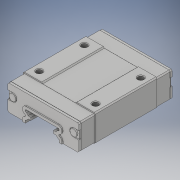
# Autodesk Inventor part: SSEBZ-MX16_b
Saved by Autodesk Inventor 2019 (Build 230136000, 136)
## iProperties
Created: 2022-12-29
Part Number: SSEBZ-MX16_b
Material: Generic
Catalog Web Link: www.cadenas.de
Description: SSEBZ, SSEBZ-MX, SSE2BZ, SSE2BZ-MX, SSEBLZ, SSEBLZ-MX, SSE2BLZ, SSE2BLZ-MX, SEBZ, SE2BZ, SEBLZ, SE2BLZ_block-Miniature Linear Guides - Standard Blocks - Light Preload/Slight Clearance - Standard Grade - Selectable/Configurable
Vendor: MISUMI
Document SubType Name: Modeling
Designer: psAdmin
Manufacturer: MISUMI
Mass: 12.2418 g
Surface Area: 52.4298 cm^2
Volume: 12.2418 cm^3
Density: 1 g/cm^3
Appearance: PSOLRGB-175-175-175
Category: PARTsolutions
Company: MISUMI
Title: SSEBZ-MX16
Author: Cadenas PARTsolutions
Comments: Miniature Linear Guides - Standard Blocks - Light Preload/Slight Clearance - Standard Grade - Selectable/Configurable
PSOL_IDENT_0: {$CADENAS_DATA/23d-libs/misumi/metric/06_linear_guides/ssebz_series/sebz_block.prj},271 {VTYP=3D},{N
PSOL_IDENT_1: B=SSEBZ-MX16_b},{LINA=SSEBZ-MX16},{NN=SSEBZ, SSEBZ-MX, SSE2BZ, SSE2BZ-MX, SSEBLZ, SSEBLZ-MX, SSE2BLZ
PSOL_IDENT_2: , SSE2BLZ-MX, SEBZ, SE2BZ, SEBLZ, SE2BLZ_block},{DATE=01.06.2021 05:33:22},{GEOMDATE=29.09.2020 01:4
PSOL_IDENT_3: 8:00},{VERSION=},{LINEID=300},{WBVAR=MAT,MX},{WBNUMERIC=}  {NB=SSEBZ-MX16_b},{LINA=SSEBZ-MX16},{KT=D
PSOL_IDENT_4: UMMY},{PN=SSEBZ-MX16},{TS=Z},{TYPE=SSEBZ},{H=16},{MAT=S},{MX=-MX},{MXALG='', 'w/o MX(Lubrication uni
PSOL_IDENT_5: t)', '-MX', 'with MX(Lubrication unit)'},{W=32},{L1=42.4},{B=25},{C=20},{SLL=M3x4},{S=3},{LL=4.0},{L
PSOL_IDENT_6: 2=27.4},{K=12.0},{CBB=0.5},{W1=15},{W2=8.5},{H1=9.5},{CAA=0.5},{F=40},{G=15.0},{CA1=0.3},{CA2=0.5},{
PSOL_IDENT_7: VA1=2.5},{HA1=2.5},{WA1=3.4477},{WA2=1.2},{RA1=3.50},{HA2=15.6300},{POIA1=0.2300},{BHA1=27.0},{BHA2=
PSOL_IDENT_8: 31.5},{BHA3=31.6},{BHA5=17.9450},{BHA6=31.1},{BHA7=14.6},{BHA8=7.4},{BVA1=5.20},{BVA3=0.50},{BVA4=0.
PSOL_IDENT_9: 60},{BVA5=11.30},{BVA6=11.40},{BCA1=0.5},{BCA2H=0.5},{BCA2V=0.45},{BRA1=1.80},{BRA2=1.50},{BDA1=25.0
PSOL_IDENT_10: 0},{BHB1=17.4600},{BHB2=15.5484},{BVB1=6.6300},{BVB2=3.5286},{BRB1=1.6},{BRB2=1.3000},{BRB3=0.4},{BH
PSOL_IDENT_11: C1=6.00},{BHC2=1.0},{BHC3=0.6},{BHC4=0.4},{BHC5=0.5},{MD=7.0}
NB: SSEBZ-MX16_b
NN: SSEBZ, SSEBZ-MX, SSE2BZ, SSE2BZ-MX, SSEBLZ, SSEBLZ-MX, SSE2BLZ, SSE2BLZ-MX, SEBZ, SE2BZ, SEBLZ, SE2BLZ_block
NT: Miniature Linear Guides - Standard Blocks - Light Preload/Slight Clearance - Standard Grade - Selectable/Configurable
NBSYN: $PN._b
LINA: SSEBZ-MX16
CATALOG: Misumi
PN: SSEBZ-MX16
H: 16
MAT: Stainless Steel
MX: with MX(Lubrication unit)
W: 32
L1: 42.4
B: 25
C: 20
SLL: M3x4
S: 3
LL: 4
L2: 27.4
K: 12
CBB: 0.5
W1: 15
W2: 8.5
H1: 9.5
CAA: 0.5
F: 40
G: 15
CA1: 0.3
CA2: 0.5
VA1: 2.5
HA1: 2.5
WA1: 3.4477
WA2: 1.2
RA1: 3.5
HA2: 15.63
POIA1: 0.23
BHA1: 27
BHA2: 31.5
BHA3: 31.6
BHA5: 17.945
BHA6: 31.1
BHA7: 14.6
BHA8: 7.4
BVA1: 5.2
BVA3: 0.5
BVA4: 0.6
BVA5: 11.3
BVA6: 11.4
BCA1: 0.5
BCA2H: 0.5
BCA2V: 0.45
BRA1: 1.8
BRA2: 1.5
BDA1: 25
BHB1: 17.46
BHB2: 15.5484
BVB1: 6.63
BVB2: 3.5286
BRB1: 1.6
BRB2: 1.3
BRB3: 0.4
BHC1: 6
BHC2: 1
BHC3: 0.6
BHC4: 0.4
BHC5: 0.5
MD: 7
SUPPLIER: MISUMI
ARTICLENO: SSEBZ-MX16_b
BOMINFO: SSEBZ-MX16
CREATOR: CADENAS GmbH
Autodesk Inventor part; units mm, degrees
sketch "Sketch_2" plane through (0, 0, 0) normal (0, 0, 1) x (1, 0, 0)
  line L0 (-16, 4.5) -> (-15.5, 4)
  line L1 (-15.5, 4) -> (-8.9725, 4)
  line L2 (-8.9725, 4) -> (-8.758, 4.1)
  line L3 (-8.758, 4.1) -> (8.758, 4.1)
  line L4 (8.758, 4.1) -> (8.9725, 4)
  line L5 (8.9725, 4) -> (15.5, 4)
  line L6 (15.5, 4) -> (16, 4.5)
  line L7 (16, 4.5) -> (16, 15.5)
  line L8 (16, 15.5) -> (15.5, 16)
  line L9 (15.5, 16) -> (7.8, 16)
  line L10 (7.8, 16) -> (7.3, 15.55)
  line L11 (7.3, 15.55) -> (-7.3, 15.55)
  line L12 (-7.3, 15.55) -> (-7.8, 16)
  line L13 (-7.8, 16) -> (-15.5, 16)
  line L14 (-15.5, 16) -> (-16, 15.5)
  line L15 (-16, 15.5) -> (-16, 4.5)
  constraints: 32 end point
extrude "Extrusion1" add sketch "Sketch_2" along normal mid plane 27.4
sketch "Sketch_3" plane through (0, 0, 13.7) normal (0, 0, 1) x (1, 0, 0)
  line L0 (-15.8, 15) -> (-15.8, 4.6)
  line L1 (-15.8, 4.6) -> (-15.3, 4.1)
  line L2 (-15.3, 4.1) -> (15.3, 4.1)
  line L3 (15.3, 4.1) -> (15.8, 4.6)
  line L4 (15.8, 4.6) -> (15.8, 15)
  line L5 (15.8, 15) -> (15.3, 15.5)
  line L6 (15.3, 15.5) -> (-15.3, 15.5)
  line L7 (-15.3, 15.5) -> (-15.8, 15)
  constraints: 16 end point
extrude "Extrusion2" add sketch "Sketch_3" along normal blind 7.5
sketch "Sketch_4" plane through (0, 0, -13.7) normal (0, 0, 1) x (1, 0, 0)
  line L0 (-15.8, 15) -> (-15.8, 4.6)
  line L1 (-15.8, 4.6) -> (-15.3, 4.1)
  line L2 (-15.3, 4.1) -> (15.3, 4.1)
  line L3 (15.3, 4.1) -> (15.8, 4.6)
  line L4 (15.8, 4.6) -> (15.8, 15)
  line L5 (15.8, 15) -> (15.3, 15.5)
  line L6 (15.3, 15.5) -> (-15.3, 15.5)
  line L7 (-15.3, 15.5) -> (-15.8, 15)
  constraints: 16 end point
extrude "Extrusion3" add sketch "Sketch_4" against normal blind 7.5
sketch "Sketch_8" plane through (0, 0, 21.2) normal (0, 0, 1) x (1, 0, 0)
  line L0 (-32, 24) -> (-32, 0)
  line L1 (-32, 0) -> (32, 0)
  line L2 (32, 0) -> (32, 24)
  line L3 (32, 24) -> (-32, 24)
  line L4 (-15.75, 12.6) -> (-13.5, 12.6)
  arc A0 (-13.5, 9) -> (-13.5, 12.6) centre (-13.5, 10.8) ccw
  line L5 (-13.5, 9) -> (-15.75, 9)
  line L6 (-15.75, 9) -> (-15.75, 4.6)
  line L7 (-15.75, 4.6) -> (-15.25, 4.1)
  line L8 (-15.25, 4.1) -> (15.25, 4.1)
  line L9 (15.25, 4.1) -> (15.75, 4.6)
  line L10 (15.75, 4.6) -> (15.75, 9)
  line L11 (15.75, 9) -> (13.5, 9)
  arc A1 (13.5, 12.6) -> (13.5, 9) centre (13.5, 10.8) ccw
  line L12 (13.5, 12.6) -> (15.75, 12.6)
  line L13 (15.75, 12.6) -> (15.75, 14.9)
  line L14 (15.75, 14.9) -> (15.25, 15.4)
  line L15 (15.25, 15.4) -> (-15.25, 15.4)
  line L16 (-15.25, 15.4) -> (-15.75, 14.9)
  line L17 (-15.75, 14.9) -> (-15.75, 12.6)
  constraints: 36 end point, 4 point on circle, 2 centre point
extrude "Extrusion4" cut sketch "Sketch_8" against normal blind 1.5
sketch "Sketch_15" plane through (0, 0, 21.2) normal (0, 0, 1) x (1, 0, 0)
  line L0 (-32, 24) -> (-32, 0)
  line L1 (-32, 0) -> (32, 0)
  line L2 (32, 0) -> (32, 24)
  line L3 (32, 24) -> (-32, 24)
  line L4 (-8.73, 4.1) -> (8.73, 4.1)
  line L5 (8.73, 4.1) -> (8.73, 5.2357)
  arc A0 (8.73, 5.2357) -> (8.0801, 6.3615) centre (7.43, 5.2357) ccw
  line L6 (8.0801, 6.3615) -> (7.5742, 6.6536)
  arc A1 (7.5742, 7.3464) -> (7.5742, 6.6536) centre (7.7742, 7) ccw
  line L7 (7.5742, 7.3464) -> (8.0801, 7.6385)
  arc A2 (8.0801, 7.6385) -> (8.73, 8.7643) centre (7.43, 8.7643) ccw
  line L8 (8.73, 8.7643) -> (8.73, 9.13)
  arc A3 (8.73, 9.13) -> (7.13, 10.73) centre (7.13, 9.13) ccw
  line L9 (7.13, 10.73) -> (-7.13, 10.73)
  arc A4 (-7.13, 10.73) -> (-8.73, 9.13) centre (-7.13, 9.13) ccw
  line L10 (-8.73, 9.13) -> (-8.73, 8.7643)
  arc A5 (-8.73, 8.7643) -> (-8.0801, 7.6385) centre (-7.43, 8.7643) ccw
  line L11 (-8.0801, 7.6385) -> (-7.5742, 7.3464)
  arc A6 (-7.5742, 6.6536) -> (-7.5742, 7.3464) centre (-7.7742, 7) ccw
  line L12 (-7.5742, 6.6536) -> (-8.0801, 6.3615)
  arc A7 (-8.0801, 6.3615) -> (-8.73, 5.2357) centre (-7.43, 5.2357) ccw
  line L13 (-8.73, 5.2357) -> (-8.73, 4.1)
  constraints: 28 end point, 16 point on circle, 8 centre point
extrude "Extrusion5" cut sketch "Sketch_15" against normal blind 0.5
sketch "Sketch_7" plane through (0, 0, -21.2) normal (0, 0, 1) x (1, 0, 0)
  line L0 (-32, 24) -> (-32, 0)
  line L1 (-32, 0) -> (32, 0)
  line L2 (32, 0) -> (32, 24)
  line L3 (32, 24) -> (-32, 24)
  line L4 (-15.75, 12.6) -> (-13.5, 12.6)
  arc A0 (-13.5, 9) -> (-13.5, 12.6) centre (-13.5, 10.8) ccw
  line L5 (-13.5, 9) -> (-15.75, 9)
  line L6 (-15.75, 9) -> (-15.75, 4.6)
  line L7 (-15.75, 4.6) -> (-15.25, 4.1)
  line L8 (-15.25, 4.1) -> (15.25, 4.1)
  line L9 (15.25, 4.1) -> (15.75, 4.6)
  line L10 (15.75, 4.6) -> (15.75, 9)
  line L11 (15.75, 9) -> (13.5, 9)
  arc A1 (13.5, 12.6) -> (13.5, 9) centre (13.5, 10.8) ccw
  line L12 (13.5, 12.6) -> (15.75, 12.6)
  line L13 (15.75, 12.6) -> (15.75, 14.9)
  line L14 (15.75, 14.9) -> (15.25, 15.4)
  line L15 (15.25, 15.4) -> (-15.25, 15.4)
  line L16 (-15.25, 15.4) -> (-15.75, 14.9)
  line L17 (-15.75, 14.9) -> (-15.75, 12.6)
  constraints: 36 end point, 4 point on circle, 2 centre point
extrude "Extrusion6" cut sketch "Sketch_7" along normal blind 1.5
sketch "Sketch_13" plane through (0, 0, -21.2) normal (0, 0, 1) x (1, 0, 0)
  line L0 (-32, 24) -> (-32, 0)
  line L1 (-32, 0) -> (32, 0)
  line L2 (32, 0) -> (32, 24)
  line L3 (32, 24) -> (-32, 24)
  line L4 (-8.73, 4.1) -> (8.73, 4.1)
  line L5 (8.73, 4.1) -> (8.73, 5.2357)
  arc A0 (8.73, 5.2357) -> (8.0801, 6.3615) centre (7.43, 5.2357) ccw
  line L6 (8.0801, 6.3615) -> (7.5742, 6.6536)
  arc A1 (7.5742, 7.3464) -> (7.5742, 6.6536) centre (7.7742, 7) ccw
  line L7 (7.5742, 7.3464) -> (8.0801, 7.6385)
  arc A2 (8.0801, 7.6385) -> (8.73, 8.7643) centre (7.43, 8.7643) ccw
  line L8 (8.73, 8.7643) -> (8.73, 9.13)
  arc A3 (8.73, 9.13) -> (7.13, 10.73) centre (7.13, 9.13) ccw
  line L9 (7.13, 10.73) -> (-7.13, 10.73)
  arc A4 (-7.13, 10.73) -> (-8.73, 9.13) centre (-7.13, 9.13) ccw
  line L10 (-8.73, 9.13) -> (-8.73, 8.7643)
  arc A5 (-8.73, 8.7643) -> (-8.0801, 7.6385) centre (-7.43, 8.7643) ccw
  line L11 (-8.0801, 7.6385) -> (-7.5742, 7.3464)
  arc A6 (-7.5742, 6.6536) -> (-7.5742, 7.3464) centre (-7.7742, 7) ccw
  line L12 (-7.5742, 6.6536) -> (-8.0801, 6.3615)
  arc A7 (-8.0801, 6.3615) -> (-8.73, 5.2357) centre (-7.43, 5.2357) ccw
  line L13 (-8.73, 5.2357) -> (-8.73, 4.1)
  constraints: 28 end point, 16 point on circle, 8 centre point
extrude "Extrusion7" cut sketch "Sketch_13" along normal blind 0.5
sketch "Sketch_25" plane through (0, 0, 19.7) normal (0, 0, 1) x (1, 0, 0)
  line L0 (-15.55, 12.6) -> (-15.55, 9)
  line L1 (-15.55, 9) -> (-13.5, 9)
  arc A0 (-13.5, 9) -> (-13.5, 12.6) centre (-13.5, 10.8) ccw
  line L2 (-13.5, 12.6) -> (-15.55, 12.6)
  constraints: 6 end point, 2 point on circle, 1 centre point
extrude "Extrusion8" add sketch "Sketch_25" along normal blind 0.6
sketch "Sketch_5" plane through (0, 0, 19.7) normal (0, 0, 1) x (1, 0, 0)
  arc A0 (13.5, 12.6) -> (13.5, 9) centre (13.5, 10.8) ccw
  line L0 (13.5, 9) -> (15.55, 9)
  line L1 (15.55, 9) -> (15.55, 12.6)
  line L2 (15.55, 12.6) -> (13.5, 12.6)
  constraints: 6 end point, 2 point on circle, 1 centre point
extrude "Extrusion9" add sketch "Sketch_5" along normal blind 0.6
sketch "Sketch_9" plane through (0, 0, -19.7) normal (0, 0, 1) x (1, 0, 0)
  line L0 (-15.55, 12.6) -> (-15.55, 9)
  line L1 (-15.55, 9) -> (-13.5, 9)
  arc A0 (-13.5, 9) -> (-13.5, 12.6) centre (-13.5, 10.8) ccw
  line L2 (-13.5, 12.6) -> (-15.55, 12.6)
  constraints: 6 end point, 2 point on circle, 1 centre point
extrude "Extrusion10" add sketch "Sketch_9" against normal blind 0.6
sketch "Sketch_26" plane through (0, 0, -19.7) normal (0, 0, 1) x (1, 0, 0)
  arc A0 (13.5, 12.6) -> (13.5, 9) centre (13.5, 10.8) ccw
  line L0 (13.5, 9) -> (15.55, 9)
  line L1 (15.55, 9) -> (15.55, 12.6)
  line L2 (15.55, 12.6) -> (13.5, 12.6)
  constraints: 6 end point, 2 point on circle, 1 centre point
extrude "Extrusion11" add sketch "Sketch_26" against normal blind 0.6
sketch "Sketch_18" plane through (-13.5, 0, 0) normal (1, 0, 0) x (0, 0, -1)
  line L0 (-20.3, 10.8) -> (-20.9, 10.8)
  line L1 (-20.9, 10.8) -> (-20.9, 12.3)
  line L2 (-20.9, 12.3) -> (-20.3, 12.3)
  line L3 (-20.3, 12.3) -> (-20.3, 10.8)
  line L4 (-20.3, 10.8) -> (-20.9, 10.8)
  constraints: 10 end point
revolve "Revolution1" add sketch "Sketch_18" angle 360 about axis through (-13.5, 10.8, 20.3) along (0, 0, -1)
sketch "Sketch_19" plane through (-13.5, 0, 0) normal (1, 0, 0) x (0, 0, -1)
  line L0 (20.9, 10.8) -> (20.3, 10.8)
  line L1 (20.3, 10.8) -> (20.3, 12.3)
  line L2 (20.3, 12.3) -> (20.9, 12.3)
  line L3 (20.9, 12.3) -> (20.9, 10.8)
  line L4 (20.9, 10.8) -> (20.3, 10.8)
  constraints: 10 end point
revolve "Revolution2" add sketch "Sketch_19" angle 360 about axis through (-13.5, 10.8, -20.9) along (0, 0, -1)
sketch "Sketch_20" plane through (13.5, 0, 0) normal (1, 0, 0) x (0, 0, -1)
  line L0 (-20.3, 10.8) -> (-20.9, 10.8)
  line L1 (-20.9, 10.8) -> (-20.9, 12.3)
  line L2 (-20.9, 12.3) -> (-20.3, 12.3)
  line L3 (-20.3, 12.3) -> (-20.3, 10.8)
  line L4 (-20.3, 10.8) -> (-20.9, 10.8)
  constraints: 10 end point
revolve "Revolution3" add sketch "Sketch_20" angle 360 about axis through (13.5, 10.8, 20.3) along (0, 0, -1)
sketch "Sketch_21" plane through (13.5, 0, 0) normal (1, 0, 0) x (0, 0, -1)
  line L0 (20.9, 10.8) -> (20.3, 10.8)
  line L1 (20.3, 10.8) -> (20.3, 12.3)
  line L2 (20.3, 12.3) -> (20.9, 12.3)
  line L3 (20.9, 12.3) -> (20.9, 10.8)
  line L4 (20.9, 10.8) -> (20.3, 10.8)
  constraints: 10 end point
revolve "Revolution4" add sketch "Sketch_21" angle 360 about axis through (13.5, 10.8, -20.9) along (0, 0, -1)
sketch "Sketch_17" plane through (0, 0, 0) normal (0, 0, 1) x (1, 0, 0)
  line L0 (-7.5, 9.2) -> (-7.5, 8.7239)
  line L1 (-7.5, 8.7239) -> (-6.94, 8.4006)
  arc A0 (-6.2177, 7.6) -> (-6.94, 8.4006) centre (-7.815, 6.885) ccw
  line L2 (-6.2177, 7.6) -> (-5, 7.6)
  line L3 (-5, 7.6) -> (-5, 6.4)
  line L4 (-5, 6.4) -> (-6.2177, 6.4)
  arc A1 (-6.94, 5.5994) -> (-6.2177, 6.4) centre (-7.815, 7.115) ccw
  line L5 (-6.94, 5.5994) -> (-7.5, 5.2762)
  line L6 (-7.5, 5.2762) -> (-7.5, 0.5)
  line L7 (-7.5, 0.5) -> (-7, 0)
  line L8 (-7, 0) -> (7, 0)
  line L9 (7, 0) -> (7.5, 0.5)
  line L10 (7.5, 0.5) -> (7.5, 5.2762)
  line L11 (7.5, 5.2762) -> (6.94, 5.5994)
  arc A2 (6.2177, 6.4) -> (6.94, 5.5994) centre (7.815, 7.115) ccw
  line L12 (6.2177, 6.4) -> (5, 6.4)
  line L13 (5, 6.4) -> (5, 7.6)
  line L14 (5, 7.6) -> (6.2177, 7.6)
  arc A3 (6.94, 8.4006) -> (6.2177, 7.6) centre (7.815, 6.885) ccw
  line L15 (6.94, 8.4006) -> (7.5, 8.7239)
  line L16 (7.5, 8.7239) -> (7.5, 9.2)
  line L17 (7.5, 9.2) -> (7.2, 9.5)
  line L18 (7.2, 9.5) -> (-7.2, 9.5)
  line L19 (-7.2, 9.5) -> (-7.5, 9.2)
  constraints: 40 end point, 8 point on circle, 4 centre point
extrude "Extrusion12" cut sketch "Sketch_17" along normal mid plane 27.4
sketch "Sketch_11" plane through (0, 0, 13.7) normal (0, 0, 1) x (1, 0, 0)
  line L0 (-7.5, 9.2) -> (-7.5, 8.7239)
  line L1 (-7.5, 8.7239) -> (-6.94, 8.4006)
  arc A0 (-6.2177, 7.6) -> (-6.94, 8.4006) centre (-7.815, 6.885) ccw
  line L2 (-6.2177, 7.6) -> (-5, 7.6)
  line L3 (-5, 7.6) -> (-5, 6.4)
  line L4 (-5, 6.4) -> (-6.2177, 6.4)
  arc A1 (-6.94, 5.5994) -> (-6.2177, 6.4) centre (-7.815, 7.115) ccw
  line L5 (-6.94, 5.5994) -> (-7.5, 5.2762)
  line L6 (-7.5, 5.2762) -> (-7.5, 0.5)
  line L7 (-7.5, 0.5) -> (-7, 0)
  line L8 (-7, 0) -> (7, 0)
  line L9 (7, 0) -> (7.5, 0.5)
  line L10 (7.5, 0.5) -> (7.5, 5.2762)
  line L11 (7.5, 5.2762) -> (6.94, 5.5994)
  arc A2 (6.2177, 6.4) -> (6.94, 5.5994) centre (7.815, 7.115) ccw
  line L12 (6.2177, 6.4) -> (5, 6.4)
  line L13 (5, 6.4) -> (5, 7.6)
  line L14 (5, 7.6) -> (6.2177, 7.6)
  arc A3 (6.94, 8.4006) -> (6.2177, 7.6) centre (7.815, 6.885) ccw
  line L15 (6.94, 8.4006) -> (7.5, 8.7239)
  line L16 (7.5, 8.7239) -> (7.5, 9.2)
  line L17 (7.5, 9.2) -> (7.2, 9.5)
  line L18 (7.2, 9.5) -> (-7.2, 9.5)
  line L19 (-7.2, 9.5) -> (-7.5, 9.2)
  constraints: 40 end point, 8 point on circle, 4 centre point
extrude "Extrusion13" cut sketch "Sketch_11" along normal blind 13.7
sketch "Sketch_22" plane through (0, 0, 13.7) normal (0, 0, 1) x (1, 0, 0)
  line L0 (-32, 24) -> (-32, 0)
  line L1 (-32, 0) -> (32, 0)
  line L2 (32, 0) -> (32, 24)
  line L3 (32, 24) -> (-32, 24)
  line L4 (-15.8, 15.05) -> (-15.8, 4.55)
  line L5 (-15.8, 4.55) -> (-15.35, 4.1)
  line L6 (-15.35, 4.1) -> (-7.55, 4.1)
  line L7 (-7.55, 4.1) -> (-7.55, 5.3262)
  line L8 (-7.55, 5.3262) -> (-7.0074, 5.6191)
  arc A0 (-7.0074, 5.6191) -> (-6.2505, 6.45) centre (-7.815, 7.115) ccw
  line L9 (-6.2505, 6.45) -> (-5.05, 6.45)
  line L10 (-5.05, 6.45) -> (-5.05, 7.55)
  line L11 (-5.05, 7.55) -> (-6.2505, 7.55)
  arc A1 (-6.2505, 7.55) -> (-7.0074, 8.3809) centre (-7.815, 6.885) ccw
  line L12 (-7.0074, 8.3809) -> (-7.55, 8.6739)
  line L13 (-7.55, 8.6739) -> (-7.55, 9.25)
  line L14 (-7.55, 9.25) -> (-7.25, 9.55)
  line L15 (-7.25, 9.55) -> (7.25, 9.55)
  line L16 (7.25, 9.55) -> (7.55, 9.25)
  line L17 (7.55, 9.25) -> (7.55, 8.6739)
  line L18 (7.55, 8.6739) -> (7.0074, 8.3809)
  arc A2 (7.0074, 8.3809) -> (6.2505, 7.55) centre (7.815, 6.885) ccw
  line L19 (6.2505, 7.55) -> (5.05, 7.55)
  line L20 (5.05, 7.55) -> (5.05, 6.45)
  line L21 (5.05, 6.45) -> (6.2505, 6.45)
  arc A3 (6.2505, 6.45) -> (7.0074, 5.6191) centre (7.815, 7.115) ccw
  line L22 (7.0074, 5.6191) -> (7.55, 5.3262)
  line L23 (7.55, 5.3262) -> (7.55, 4.1)
  line L24 (7.55, 4.1) -> (15.35, 4.1)
  line L25 (15.35, 4.1) -> (15.8, 4.55)
  line L26 (15.8, 4.55) -> (15.8, 15.05)
  line L27 (15.8, 15.05) -> (15.35, 15.5)
  line L28 (15.35, 15.5) -> (-15.35, 15.5)
  line L29 (-15.35, 15.5) -> (-15.8, 15.05)
  constraints: 60 end point, 8 point on circle, 4 centre point
extrude "Extrusion14" cut sketch "Sketch_22" along normal blind 0.05
sketch "Sketch_10" plane through (0, 0, -13.7) normal (0, 0, 1) x (1, 0, 0)
  line L0 (-7.5, 9.2) -> (-7.5, 8.7239)
  line L1 (-7.5, 8.7239) -> (-6.94, 8.4006)
  arc A0 (-6.2177, 7.6) -> (-6.94, 8.4006) centre (-7.815, 6.885) ccw
  line L2 (-6.2177, 7.6) -> (-5, 7.6)
  line L3 (-5, 7.6) -> (-5, 6.4)
  line L4 (-5, 6.4) -> (-6.2177, 6.4)
  arc A1 (-6.94, 5.5994) -> (-6.2177, 6.4) centre (-7.815, 7.115) ccw
  line L5 (-6.94, 5.5994) -> (-7.5, 5.2762)
  line L6 (-7.5, 5.2762) -> (-7.5, 0.5)
  line L7 (-7.5, 0.5) -> (-7, 0)
  line L8 (-7, 0) -> (7, 0)
  line L9 (7, 0) -> (7.5, 0.5)
  line L10 (7.5, 0.5) -> (7.5, 5.2762)
  line L11 (7.5, 5.2762) -> (6.94, 5.5994)
  arc A2 (6.2177, 6.4) -> (6.94, 5.5994) centre (7.815, 7.115) ccw
  line L12 (6.2177, 6.4) -> (5, 6.4)
  line L13 (5, 6.4) -> (5, 7.6)
  line L14 (5, 7.6) -> (6.2177, 7.6)
  arc A3 (6.94, 8.4006) -> (6.2177, 7.6) centre (7.815, 6.885) ccw
  line L15 (6.94, 8.4006) -> (7.5, 8.7239)
  line L16 (7.5, 8.7239) -> (7.5, 9.2)
  line L17 (7.5, 9.2) -> (7.2, 9.5)
  line L18 (7.2, 9.5) -> (-7.2, 9.5)
  line L19 (-7.2, 9.5) -> (-7.5, 9.2)
  constraints: 40 end point, 8 point on circle, 4 centre point
extrude "Extrusion15" cut sketch "Sketch_10" against normal blind 13.7
sketch "Sketch_23" plane through (0, 0, -13.7) normal (0, 0, 1) x (1, 0, 0)
  line L0 (-32, 24) -> (-32, 0)
  line L1 (-32, 0) -> (32, 0)
  line L2 (32, 0) -> (32, 24)
  line L3 (32, 24) -> (-32, 24)
  line L4 (-15.8, 15.05) -> (-15.8, 4.55)
  line L5 (-15.8, 4.55) -> (-15.35, 4.1)
  line L6 (-15.35, 4.1) -> (-7.55, 4.1)
  line L7 (-7.55, 4.1) -> (-7.55, 5.3262)
  line L8 (-7.55, 5.3262) -> (-7.0074, 5.6191)
  arc A0 (-7.0074, 5.6191) -> (-6.2505, 6.45) centre (-7.815, 7.115) ccw
  line L9 (-6.2505, 6.45) -> (-5.05, 6.45)
  line L10 (-5.05, 6.45) -> (-5.05, 7.55)
  line L11 (-5.05, 7.55) -> (-6.2505, 7.55)
  arc A1 (-6.2505, 7.55) -> (-7.0074, 8.3809) centre (-7.815, 6.885) ccw
  line L12 (-7.0074, 8.3809) -> (-7.55, 8.6739)
  line L13 (-7.55, 8.6739) -> (-7.55, 9.25)
  line L14 (-7.55, 9.25) -> (-7.25, 9.55)
  line L15 (-7.25, 9.55) -> (7.25, 9.55)
  line L16 (7.25, 9.55) -> (7.55, 9.25)
  line L17 (7.55, 9.25) -> (7.55, 8.6739)
  line L18 (7.55, 8.6739) -> (7.0074, 8.3809)
  arc A2 (7.0074, 8.3809) -> (6.2505, 7.55) centre (7.815, 6.885) ccw
  line L19 (6.2505, 7.55) -> (5.05, 7.55)
  line L20 (5.05, 7.55) -> (5.05, 6.45)
  line L21 (5.05, 6.45) -> (6.2505, 6.45)
  arc A3 (6.2505, 6.45) -> (7.0074, 5.6191) centre (7.815, 7.115) ccw
  line L22 (7.0074, 5.6191) -> (7.55, 5.3262)
  line L23 (7.55, 5.3262) -> (7.55, 4.1)
  line L24 (7.55, 4.1) -> (15.35, 4.1)
  line L25 (15.35, 4.1) -> (15.8, 4.55)
  line L26 (15.8, 4.55) -> (15.8, 15.05)
  line L27 (15.8, 15.05) -> (15.35, 15.5)
  line L28 (15.35, 15.5) -> (-15.35, 15.5)
  line L29 (-15.35, 15.5) -> (-15.8, 15.05)
  constraints: 60 end point, 8 point on circle, 4 centre point
extrude "Extrusion16" cut sketch "Sketch_23" against normal blind 0.05
sketch "Sketch21" plane through (-15.5, 16, 13.7) normal (0, 1, 0) x (1, 0, 0)
  point P0 (3, 23.7)
hole "Hole1" at (-12.5, 16, -10) direction (0, -1, 0) diameter 2.459 depth 7 tip angle 120 countersink diameter 3 countersink angle 90 thread size "M3x0.5" class "6H" standard "ISO Metric profile"
pattern_linear "Rectangular Pattern1" count 2 spacing 25 along (1, 0, 0) count 2 spacing 20 along (0, 0, 1) of "Hole1"
ref_plane "to_rail_XY" through (0, 9.5, 0) normal (0, 0, -1) x (1, 0, 0)
ref_plane "to_rail_YZ" through (0, 9.5, 0) normal (1, 0, 0) x (0, -1, 0)
ref_plane "to_rail_ZX" through (0, 9.5, 0) normal (0, -1, 0) x (0, 0, -1)
body "Solid1"
